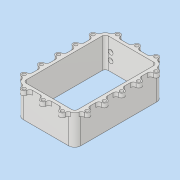
# Autodesk Inventor part: BatteryCaseSide1
Saved by Autodesk Inventor 2017 (Build 210142000, 142)
## iProperties
Created: 2018-02-14
Part Number: BatteryCaseSide1
Material: ABS Plastic
Document SubType Name: Modeling
Designer: Derek Wider
Density: 1.06 g/cm^3
Appearance: Smooth - White
Author: Derek Wider
Autodesk Inventor part; units mm, degrees
ref_plane "YZ Plane" through (0, 0, 0) normal (1, 0, 0) x (0, 1, 0)
ref_plane "XZ Plane" through (0, 0, 0) normal (0, 1, 0) x (-1, 0, 0)
ref_plane "XY Plane" through (0, 0, 0) normal (0, 0, 1) x (1, 0, 0)
sketch "Sketch1" plane through (0, 0, 0) normal (0, 1, 0) x (-1, 0, 0)
  line L0 (4.7625, 0) -> (53.0225, 0)
  line L1 (57.785, -4.7625) -> (57.785, -85.4075)
  line L2 (53.0225, -90.17) -> (4.7625, -90.17)
  line L3 (0, -85.4075) -> (0, -4.7625)
  arc A0 (57.785, -4.7625) -> (53.0225, 0) centre (53.0225, -4.7625) ccw
  arc A1 (4.7625, 0) -> (0, -4.7625) centre (4.7625, -4.7625) ccw
  arc A2 (0, -85.4075) -> (4.7625, -90.17) centre (4.7625, -85.4075) ccw
  arc A3 (53.0225, -90.17) -> (57.785, -85.4075) centre (53.0225, -85.4075) ccw
  line L4 (56.1975, -85.4075) -> (56.1975, -4.7625)
  arc A4 (56.1975, -4.7625) -> (53.0225, -1.5875) centre (53.0225, -4.7625) ccw
  line L5 (53.0225, -1.5875) -> (4.7625, -1.5875)
  arc A5 (4.7625, -1.5875) -> (1.5875, -4.7625) centre (4.7625, -4.7625) ccw
  line L6 (1.5875, -4.7625) -> (1.5875, -85.4075)
  arc A6 (1.5875, -85.4075) -> (4.7625, -88.5825) centre (4.7625, -85.4075) ccw
  line L7 (4.7625, -88.5825) -> (53.0225, -88.5825)
  arc A7 (53.0225, -88.5825) -> (56.1975, -85.4075) centre (53.0225, -85.4075) ccw
  line L8 (59.3725, -85.4075) -> (59.3725, -4.7625)
  arc A8 (59.3725, -4.7625) -> (53.0225, 1.5875) centre (53.0225, -4.7625) ccw
  line L9 (53.0225, 1.5875) -> (4.7625, 1.5875)
  arc A9 (4.7625, 1.5875) -> (-1.5875, -4.7625) centre (4.7625, -4.7625) ccw
  line L10 (-1.5875, -4.7625) -> (-1.5875, -85.4075)
  arc A10 (-1.5875, -85.4075) -> (4.7625, -91.7575) centre (4.7625, -85.4075) ccw
  line L11 (4.7625, -91.7575) -> (53.0225, -91.7575)
  arc A11 (53.0225, -91.7575) -> (59.3725, -85.4075) centre (53.0225, -85.4075) ccw
  point P0 (0, 0)
  point P1 (57.785, -90.17)
  point P2 (57.785, 0)
  point P3 (0, -90.17)
  dimension "d0" = 90.17
  dimension "d1" = 57.785
  dimension "d2" = 4.7625
  dimension "d3" = 1.5875
  dimension "d4" = 1.5875
  constraints: 24 end point, 24 point on circle, 12 centre point, 8 point on line, 8 tangent, 6 parallel, 3 equal radius, 3 perpendicular, 1 horizontal, 14 other
  measures "d0" distance of point (57.785, 0) point (57.785, -90.17)
  measures "d1" distance of point (57.785, -90.17) point (0, -90.17)
  measures "d2" radius of A0
  measures "d3" distance between parallel lines of L1 L4
  measures "d4" distance between parallel lines of L1 L8
extrude "Extrusion1" add sketch "Sketch1" along normal blind 31.75 contours L0 A0 L1 A3 L2 A2 L3 A1 | A11 L11 A10 L10 A9 L9 A8 L8
sketch "Sketch2" plane through (0, 31.75, 0) normal (0, 1, 0) x (1, 0, 0)
  line L0 (1.5875, 4.7625) -> (1.5875, 85.4075) construction
  arc A0 (1.5875, 85.4075) -> (-4.7625, 91.7575) centre (-4.7625, 85.4075) ccw construction
  line L1 (-4.7625, 91.7575) -> (-53.0225, 91.7575) construction
  arc A1 (-53.0225, 91.7575) -> (-59.3725, 85.4075) centre (-53.0225, 85.4075) ccw construction
  line L2 (-59.3725, 85.4075) -> (-59.3725, 4.7625) construction
  arc A2 (-59.3725, 4.7625) -> (-53.0225, -1.5875) centre (-53.0225, 4.7625) ccw construction
  line L3 (-53.0225, -1.5875) -> (-4.7625, -1.5875) construction
  arc A3 (-4.7625, -1.5875) -> (1.5875, 4.7625) centre (-4.7625, 4.7625) ccw construction
  circle A4 centre (-49.2125, 94.6785) radius 1.778
  circle A5 centre (-49.2125, 94.6785) radius 2.921
  circle A6 centre (-28.8925, 94.6785) radius 1.778
  circle A7 centre (-28.8925, 94.6785) radius 2.921
  circle A8 centre (-62.2935, 81.5975) radius 1.778
  circle A9 centre (-62.2935, 81.5975) radius 2.921
  circle A10 centre (-62.2935, 63.3412) radius 1.778
  circle A11 centre (-62.2935, 63.3412) radius 2.921
  line L4 (-28.8925, 94.6785) -> (-28.8925, 104.7777) construction
  circle A12 centre (-62.2935, 45.085) radius 1.778
  circle A13 centre (-62.2935, 45.085) radius 2.921
  circle A14 centre (-62.2935, 26.8288) radius 1.778
  circle A15 centre (-62.2935, 26.8288) radius 2.921
  circle A16 centre (-62.2935, 8.5725) radius 1.778
  circle A17 centre (-62.2935, 8.5725) radius 2.921
  circle A18 centre (-49.2125, -4.5085) radius 1.778
  circle A19 centre (-49.2125, -4.5085) radius 2.921
  circle A20 centre (-28.8925, -4.5085) radius 1.778
  circle A21 centre (-28.8925, -4.5085) radius 2.921
  line L5 (-46.2915, 94.6785) -> (-46.2915, 91.7575)
  line L6 (-4.7625, 91.7575) -> (-53.0225, 91.7575) projected
  line L7 (-52.1335, 94.6785) -> (-52.1335, 91.7575)
  line L8 (-62.2935, 84.5185) -> (-59.3725, 84.5185)
  line L9 (-62.2935, 78.6765) -> (-59.3725, 78.6765)
  line L10 (-59.3725, 84.5185) -> (-59.3725, 78.6765)
  line L11 (-62.2935, 66.2623) -> (-59.3725, 66.2622)
  line L12 (-62.2935, 60.4202) -> (-59.3725, 60.4202)
  line L13 (-59.3725, 66.2622) -> (-59.3725, 60.4202)
  line L14 (-62.2935, 48.006) -> (-59.3725, 48.006)
  line L15 (-62.2935, 42.164) -> (-59.3725, 42.164)
  line L16 (-59.3725, 48.006) -> (-59.3725, 42.164)
  line L17 (-62.2935, 29.7498) -> (-59.3725, 29.7498)
  line L18 (-62.2935, 23.9078) -> (-59.3725, 23.9078)
  line L19 (-59.3725, 29.7498) -> (-59.3725, 23.9078)
  line L20 (-62.2935, 11.4935) -> (-59.3725, 11.4935)
  line L21 (-62.2935, 5.6515) -> (-59.3725, 5.6515)
  line L22 (-59.3725, 5.6515) -> (-59.3725, 11.4935)
  line L23 (-46.2915, -4.5085) -> (-46.2915, -1.5875)
  line L24 (-52.1335, -4.5085) -> (-52.1335, -1.5875)
  line L25 (-46.2915, -1.5875) -> (-52.1335, -1.5875)
  line L26 (-25.9715, -4.5085) -> (-25.9715, -1.5875)
  line L27 (-31.8135, -4.5085) -> (-31.8135, -1.5875)
  line L28 (-31.8135, -1.5875) -> (-25.9715, -1.5875)
  line L29 (-31.8135, 94.6785) -> (-31.8135, 91.7575)
  line L30 (-25.9715, 94.6785) -> (-25.9715, 91.7575)
  line L31 (-31.8135, 91.7575) -> (-25.9715, 91.7575)
  line L32 (-46.2915, 91.7575) -> (-52.1335, 91.7575)
  line L33 (-53.0225, 91.7575) -> (-4.7625, 91.7575) construction
  arc A22 (1.5875, 85.4075) -> (-4.7625, 91.7575) centre (-4.7625, 85.4075) ccw construction
  line L34 (1.5875, 85.4075) -> (1.5875, 4.7625) construction
  line L35 (-4.7625, -1.5875) -> (-53.0225, -1.5875) construction
  circle A23 centre (-8.5725, 94.6785) radius 1.778
  circle A24 centre (-8.5725, 94.6785) radius 2.921
  circle A25 centre (4.5085, 81.5975) radius 1.778
  circle A26 centre (4.5085, 81.5975) radius 2.921
  circle A27 centre (4.5085, 63.3412) radius 1.778
  circle A28 centre (4.5085, 63.3412) radius 2.921
  circle A29 centre (4.5085, 45.085) radius 1.778
  circle A30 centre (4.5085, 45.085) radius 2.921
  circle A31 centre (4.5085, 26.8288) radius 1.778
  circle A32 centre (4.5085, 26.8288) radius 2.921
  circle A33 centre (4.5085, 8.5725) radius 1.778
  circle A34 centre (4.5085, 8.5725) radius 2.921
  circle A35 centre (-8.5725, -4.5085) radius 1.778
  circle A36 centre (-8.5725, -4.5085) radius 2.921
  line L36 (-11.4935, 94.6785) -> (-11.4935, 91.7575)
  line L37 (-53.0225, 91.7575) -> (-4.7625, 91.7575)
  line L38 (-5.6515, 94.6785) -> (-5.6515, 91.7575)
  line L39 (4.5085, 84.5185) -> (1.5875, 84.5185)
  line L40 (4.5085, 78.6765) -> (1.5875, 78.6765)
  line L41 (1.5875, 84.5185) -> (1.5875, 78.6765)
  line L42 (4.5085, 66.2623) -> (1.5875, 66.2622)
  line L43 (4.5085, 60.4202) -> (1.5875, 60.4202)
  line L44 (1.5875, 66.2622) -> (1.5875, 60.4202)
  line L45 (4.5085, 48.006) -> (1.5875, 48.006)
  line L46 (4.5085, 42.164) -> (1.5875, 42.164)
  line L47 (1.5875, 48.006) -> (1.5875, 42.164)
  line L48 (4.5085, 29.7498) -> (1.5875, 29.7498)
  line L49 (4.5085, 23.9078) -> (1.5875, 23.9078)
  line L50 (1.5875, 29.7498) -> (1.5875, 23.9078)
  line L51 (4.5085, 11.4935) -> (1.5875, 11.4935)
  line L52 (4.5085, 5.6515) -> (1.5875, 5.6515)
  line L53 (1.5875, 5.6515) -> (1.5875, 11.4935)
  line L54 (-11.4935, -4.5085) -> (-11.4935, -1.5875)
  line L55 (-5.6515, -4.5085) -> (-5.6515, -1.5875)
  line L56 (-11.4935, -1.5875) -> (-5.6515, -1.5875)
  line L57 (-11.4935, 91.7575) -> (-5.6515, 91.7575)
  point P0 (0, 0)
  dimension "d9" = 3.556
  dimension "d10" = 5.842
  dimension "d12" = 10.16
  dimension "d14" = 10.16
  dimension "d15" = 18.2563
  dimension "d16" = 10.16
  dimension "d17" = 18.2563
  dimension "d18" = 18.2563
  dimension "d19" = 10.16
  constraints: 104 end point, 47 symmetric about line, 34 point on circle, 33 centre point, 19 tangent, 16 coincident, 16 equal radius, 16 point on line, 10 perpendicular, 8 horizontal, 5 vertical, 3 collinear, 43 other
  measures "d9" diameter of A4
  measures "d10" diameter of A5
  measures "d14" distance from line of A8.centre L1
  measures "d15" distance of A9.centre A10.centre
  measures "d16" distance from line of L3 A16.centre
  measures "d17" distance of A16.centre A14.centre
  measures "d18" distance of A14.centre A12.centre
extrude "Extrusion3" add sketch "Sketch2" against normal blind 4.445
fillet "Fillet1" radius 3.175 32 edges at (-5.6515, 29.5275, 1.5875) (1.5875, 29.5275, -5.6515) (1.5875, 29.5275, -11.4935) (1.5875, 29.5275, -23.9078) (1.5875, 29.5275, -29.7498) (1.5875, 29.5275, -42.164) (1.5875, 29.5275, -48.006) (1.5875, 29.5275, -60.4202) (1.5875, 29.5275, -66.2622) (1.5875, 29.5275, -78.6765) (1.5875, 29.5275, -84.5185) (-5.6515, 29.5275, -91.7575) (-11.4935, 29.5275, -91.7575) (-25.9715, 29.5275, -91.7575) (-31.8135, 29.5275, -91.7575) (-46.2915, 29.5275, -91.7575) (-52.1335, 29.5275, -91.7575) (-59.3725, 29.5275, -84.5185) (-59.3725, 29.5275, -78.6765) (-59.3725, 29.5275, -66.2622) (-59.3725, 29.5275, -60.4202) (-59.3725, 29.5275, -48.006) (-59.3725, 29.5275, -42.164) (-59.3725, 29.5275, -29.7498) (-59.3725, 29.5275, -23.9078) (-59.3725, 29.5275, -11.4935) (-59.3725, 29.5275, -5.6515) (-52.1335, 29.5275, 1.5875) (-46.2915, 29.5275, 1.5875) (-25.9715, 29.5275, 1.5875) (-31.8135, 29.5275, 1.5875) (-11.4935, 29.5275, 1.5875)
sketch "Sketch4" plane through (-4.7625, 0, -91.7575) normal (0, 0, -1) x (-1, 0, 0)
  circle A0 centre (45.72, 18.034) radius 2.54
  circle A1 centre (45.72, 10.16) radius 2.54
  line L0 (0, 0) -> (48.26, 0) projected
  line L1 (48.26, 0) -> (48.26, 27.305) projected
  point P0 (-4.7625, 0)
  dimension "d29" = 7.874
  dimension "d30" = 10.16
  dimension "d31" = 5.08
  constraints: 2 centre point, 1 equal radius, 1 tangent, 1 vertical alignment
  measures "d29" distance of A1.centre A0.centre
  measures "d30" distance from line of L0 A1.centre
  measures "d31" diameter of A0
extrude "Extrusion5" cut sketch "Sketch4" against normal blind 25.4
equation "\"d3\" = d4"
equation "\"d17\" = d18"
equation "\"d18\" = d15"
equation "\"d19\" = d12"
body "Solid1"
